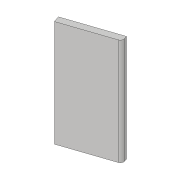
# Autodesk Inventor part: Lidar Sensor Case Piece 4
Saved by Autodesk Inventor 2018.3 (Build 223284000, 284)
## iProperties
Created: 2019-02-26
Part Number: Lidar Sensor Case Piece 4
Material: Generic
Document SubType Name: Modeling
Designer: aye06091
Mass: 3.54131 g
Surface Area: 28.2144 cm^2
Volume: 3.54131 cm^3
Density: 1 g/cm^3
Appearance: Default
Author: aye06091
Autodesk Inventor part; units mm, degrees
ref_plane "YZ Plane" through (0, 0, 0) normal (1, 0, 0) x (0, 1, 0)
ref_plane "XZ Plane" through (0, 0, 0) normal (0, 1, 0) x (-1, 0, 0)
ref_plane "XY Plane" through (0, 0, 0) normal (0, 0, 1) x (1, 0, 0)
sketch "Sketch1" plane through (0, 0, 0) normal (0, 1, 0) x (-1, 0, 0)
  line L0 (-1.958, 8.8218) -> (-25.4378, 0.9475)
  line L1 (-26.3747, 3.741) -> (-2.8949, 11.6153)
  line L2 (-1.958, 8.8218) -> (-2.8949, 11.6153)
  line L3 (-25.4378, 0.9475) -> (-26.3747, 3.741)
  point P0 (0, 0)
  point P1 (-9.2456, 5.0352)
  dimension "d0" = 24.765
  dimension "d5" = 2.9464
  constraints: 8 end point
  measures "d0" distance of L0.start L0.end
  measures "d5" distance between parallel lines of L1 L0
extrude "Extrusion1" add sketch "Sketch1" along normal blind 48.895
fillet "Fillet1" radius 1.5875 1 edges at (26.3747, 24.4475, 3.741)
body "Solid1"
